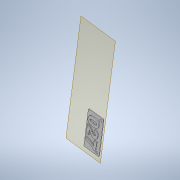
# Autodesk Inventor part: ID Plate
Saved by Autodesk Inventor 2020 (Build 240168000, 168)
## iProperties
Created: 2019-12-31
Part Number: ID Plate
Material: Generic
Document SubType Name: Modeling
Designer: pepd9
Density: 1 g/cm^3
Appearance: Default
Mass: 1.63968 g
Surface Area: 27.9863 cm^2
Volume: 1.63968 cm^3
Author: pepd9
Autodesk Inventor part; units mm, degrees
ref_plane "YZ Plane" through (0, 0, 0) normal (1, 0, 0) x (0, 1, 0)
ref_plane "XZ Plane" through (0, 0, 0) normal (0, 1, 0) x (-1, 0, 0)
ref_plane "XY Plane" through (0, 0, 0) normal (0, 0, 1) x (1, 0, 0)
ref_plane "Work Plane1" through (6.35, -3.5793, 0) normal (0, 0, 1) x (0.9913632, -0.1311451, 0)
sketch "Sketch1" plane through (6.35, -3.5793, 0) normal (0, 0, 1) x (0.9913632, -0.1311451, 0)
  line L0 (9.4349, -35.1273) -> (9.1077, -32.6537) projected
  line L1 (9.1077, -32.6537) -> (11.809, -32.2963) projected
  line L2 (11.809, -32.2963) -> (11.8581, -32.8269) projected
  line L3 (11.8581, -32.8269) -> (12.0044, -33.5342) projected
  spline S0 degree 2 poles (12.0044, -33.5342) (12.2496, -34.5127) (12.9939, -35.3621) (13.7166, -35.5719) knots 0 0 0 1 2 2 2 projected
  line L4 (13.7166, -35.5719) -> (14.274, -35.6456) projected
  line L5 (14.274, -35.6456) -> (14.6409, -38.4193) projected
  line L6 (14.6409, -38.4193) -> (0.7619, -40.2553) projected
  line L7 (0.7619, -40.2553) -> (0.2443, -36.3431) projected
  line L8 (0.2443, -36.3431) -> (9.4349, -35.1273) projected
  line L9 (-0.9482, -27.3284) -> (-1.4726, -23.3645) projected
  line L10 (-1.4726, -23.3645) -> (12.4065, -21.5284) projected
  line L11 (12.4065, -21.5284) -> (13.1225, -26.9414) projected
  spline S1 degree 2 poles (13.1225, -26.9414) (13.3717, -28.825) (11.9849, -30.9988) (10.2534, -31.5228) knots 0 0 0 1 2 2 2 projected
  spline S2 degree 2 poles (10.2534, -31.5228) (9.6848, -31.6822) (9.2839, -31.7563) (9.1286, -31.7769) knots 0 0 0 1 2 2 2 projected
  spline S3 degree 2 poles (9.1286, -31.7769) (7.1725, -32.0356) (4.658, -29.904) (4.3718, -27.7409) knots 0 0 0 1 2 2 2 projected
  line L12 (4.3718, -27.7409) -> (4.2267, -26.6439) projected
  line L13 (4.2267, -26.6439) -> (-0.9482, -27.3284) projected
  line L14 (-4.2533, -2.344) -> (-4.7325, 1.2784) projected
  line L15 (-4.7325, 1.2784) -> (9.1465, 3.1145) projected
  line L16 (9.1465, 3.1145) -> (9.8448, -2.1639) projected
  line L17 (9.8448, -2.1639) -> (2.0845, -4.5596) projected
  line L18 (2.0845, -4.5596) -> (10.2008, -4.8549) projected
  line L19 (10.2008, -4.8549) -> (10.9018, -10.154) projected
  line L20 (10.9018, -10.154) -> (-2.9773, -11.99) projected
  line L21 (-2.9773, -11.99) -> (-3.4565, -8.3676) projected
  line L22 (-3.4565, -8.3676) -> (6.1067, -7.1025) projected
  line L23 (6.1067, -7.1025) -> (-3.6564, -6.8565) projected
  line L24 (-3.6564, -6.8565) -> (-4.0562, -3.8344) projected
  line L25 (-4.0562, -3.8344) -> (5.3099, -1.0789) projected
  line L26 (5.3099, -1.0789) -> (-4.2533, -2.344) projected
  line L27 (-6.2934, 13.0772) -> (-6.8178, 17.0412) projected
  line L28 (-6.8178, 17.0412) -> (7.0613, 18.8772) projected
  line L29 (7.0613, 18.8772) -> (7.7774, 13.4643) projected
  spline S4 degree 2 poles (7.7774, 13.4643) (8.0266, 11.5806) (6.6397, 9.4068) (4.9082, 8.8829) knots 0 0 0 1 2 2 2 projected
  spline S5 degree 2 poles (4.9082, 8.8829) (4.3396, 8.7234) (3.9387, 8.6493) (3.7835, 8.6288) knots 0 0 0 1 2 2 2 projected
  spline S6 degree 2 poles (3.7835, 8.6288) (1.8273, 8.37) (-0.6872, 10.5016) (-0.9734, 12.6647) knots 0 0 0 1 2 2 2 projected
  line L30 (-0.9734, 12.6647) -> (-1.1185, 13.7618) projected
  line L31 (-1.1185, 13.7618) -> (-6.2934, 13.0772) projected
  line L32 (-8.8852, 32.6694) -> (-9.4096, 36.6333) projected
  line L33 (-9.4096, 36.6333) -> (4.4695, 38.4694) projected
  line L34 (4.4695, 38.4694) -> (5.1856, 33.0564) projected
  spline S7 degree 2 poles (5.1856, 33.0564) (5.4348, 31.1728) (4.0479, 28.999) (2.3164, 28.475) knots 0 0 0 1 2 2 2 projected
  spline S8 degree 2 poles (2.3164, 28.475) (1.7478, 28.3156) (1.3469, 28.2415) (1.1917, 28.2209) knots 0 0 0 1 2 2 2 projected
  spline S9 degree 2 poles (1.1917, 28.2209) (-0.7645, 27.9622) (-3.279, 30.0938) (-3.5652, 32.2569) knots 0 0 0 1 2 2 2 projected
  line L35 (-3.5652, 32.2569) -> (-3.7103, 33.3539) projected
  line L36 (-3.7103, 33.3539) -> (-8.8852, 32.6694) projected
  line L37 (-6.9369, 17.9416) -> (-8.0596, 26.4284) projected
  line L38 (-8.0596, 26.4284) -> (5.8195, 28.2645) projected
  line L39 (5.8195, 28.2645) -> (6.923, 19.9225) projected
  line L40 (6.923, 19.9225) -> (3.7146, 19.4981) projected
  line L41 (3.7146, 19.4981) -> (3.1354, 23.8761) projected
  line L42 (3.1354, 23.8761) -> (1.0655, 23.6022) projected
  line L43 (1.0655, 23.6022) -> (1.609, 19.4934) projected
  line L44 (1.609, 19.4934) -> (-1.4649, 19.0867) projected
  line L45 (-1.4649, 19.0867) -> (-2.0084, 23.1956) projected
  line L46 (-2.0084, 23.1956) -> (-4.3268, 22.8889) projected
  line L47 (-4.3268, 22.8889) -> (-3.7284, 18.366) projected
  line L48 (-3.7284, 18.366) -> (-6.9369, 17.9416) projected
  line L49 (-2.3023, -17.0925) -> (-2.7993, -13.3355) projected
  line L50 (-2.7993, -13.3355) -> (11.0798, -11.4995) projected
  line L51 (11.0798, -11.4995) -> (11.5768, -15.2564) projected
  line L52 (11.5768, -15.2564) -> (4.8598, -16.145) projected
  line L53 (4.8598, -16.145) -> (8.406, -17.3187) projected
  line L54 (8.406, -17.3187) -> (8.9249, -21.2413) projected
  line L55 (8.9249, -21.2413) -> (4.2393, -19.0178) projected
  line L56 (4.2393, -19.0178) -> (-1.5205, -23.0022) projected
  line L57 (-1.5205, -23.0022) -> (-2.0504, -18.9968) projected
  line L58 (-2.0504, -18.9968) -> (1.2432, -16.9078) projected
  line L59 (1.2432, -16.9078) -> (0.4818, -16.7242) projected
  line L60 (0.4818, -16.7242) -> (-2.3023, -17.0925) projected
  line L61 (20, -51) -> (-3, -51)
  line L62 (-3, -51) -> (-3, -104)
  line L63 (-3, -104) -> (20, -104)
  line L64 (20, -104) -> (20, -51)
  circle A0 centre (16.3103, -49.711) radius 1.95 projected
  circle A1 centre (-20.0656, -79.7409) radius 1.95 projected
  circle A2 centre (-37.1145, 49.1363) radius 1.95 projected
  line L65 (11.0027, -81.1536) -> (12.4808, -77.5789) projected
  line L66 (7.1679, -81.6609) -> (11.0027, -81.1536) projected
  line L67 (4.8111, -78.5935) -> (7.1679, -81.6609) projected
  line L68 (6.2892, -75.0188) -> (4.8111, -78.5935) projected
  line L69 (10.124, -74.5115) -> (6.2892, -75.0188) projected
  line L70 (12.4808, -77.5789) -> (10.124, -74.5115) projected
  line L71 (2.8138, -48.7477) -> (1.3358, -52.3224) projected
  line L72 (6.6487, -48.2404) -> (2.8138, -48.7477) projected
  line L73 (9.0054, -51.3078) -> (6.6487, -48.2404) projected
  line L74 (7.5273, -54.8825) -> (9.0054, -51.3078) projected
  line L75 (3.6925, -55.3898) -> (7.5273, -54.8825) projected
  line L76 (1.3358, -52.3224) -> (3.6925, -55.3898) projected
  line L77 (9.7896, -71.9835) -> (11.2677, -68.4088) projected
  line L78 (5.9548, -72.4908) -> (9.7896, -71.9835) projected
  line L79 (3.598, -69.4234) -> (5.9548, -72.4908) projected
  line L80 (5.0761, -65.8487) -> (3.598, -69.4234) projected
  line L81 (8.9109, -65.3414) -> (5.0761, -65.8487) projected
  line L82 (11.2677, -68.4088) -> (8.9109, -65.3414) projected
  line L83 (8.5514, -92.1198) -> (7.0733, -95.6945) projected
  line L84 (12.3863, -91.6125) -> (8.5514, -92.1198) projected
  line L85 (14.743, -94.6799) -> (12.3863, -91.6125) projected
  line L86 (13.2649, -98.2547) -> (14.743, -94.6799) projected
  line L87 (9.4301, -98.762) -> (13.2649, -98.2547) projected
  line L88 (7.0733, -95.6945) -> (9.4301, -98.762) projected
  circle A3 centre (-24, -50) radius 1.95 projected
  line L89 (-23.7833, -80.2327) -> (-27.715, -50.5115) projected
  arc A4 (-23.7833, -80.2327) -> (-21.1747, -83.3231) centre (-20.0656, -79.7409) ccw projected
  line L90 (7.3797, -99.9093) -> (-21.1747, -83.3231) projected
  arc A5 (7.3797, -99.9093) -> (7.8548, -100.0043) centre (7.7565, -99.2608) ccw projected
  line L91 (25.6777, -97.6465) -> (7.8548, -100.0043) projected
  arc A6 (25.6777, -97.6465) -> (26.3228, -96.8047) centre (25.5793, -96.903) ccw projected
  line L92 (8.768, 35.8971) -> (26.3228, -96.8047) projected
  arc A7 (8.768, 35.8971) -> (5.0328, 42.3573) centre (-0.8978, 34.6184) ccw projected
  line L93 (-5.2293, 50.2216) -> (5.0328, 42.3573) projected
  arc A8 (-5.2293, 50.2216) -> (-12.4386, 52.1485) centre (-11.1599, 42.4827) ccw projected
  line L94 (-13.3095, 52.0332) -> (-12.4386, 52.1485) projected
  line L95 (-37.6265, 52.8512) -> (-13.3095, 52.0332) projected
  arc A9 (-37.6265, 52.8512) -> (-40.8346, 48.6639) centre (-37.1145, 49.1363) ccw projected
  line L96 (-26.3408, 0.1259) -> (-40.8346, 48.6639) projected
  line L97 (-27.715, -50.5115) -> (-26.3408, 0.1259) projected
  circle A10 centre (22.2118, -94.3224) radius 1.95 projected
  point P0 (-6.7645, 2.7156)
  point P1 (1.0219, -104)
  point P2 (20, -103)
  dimension "d0" = 23
  dimension "d1" = 53
  constraints: 8 end point, 2 parallel, 2 point on line, 1 horizontal, 1 perpendicular
  measures "d0" distance of L62.end L63.end
  measures "d1" distance of L63.end L61.start
extrude "Extrusion1" add sketch "Sketch1" along normal blind 1 contours L64 L91 A5 L90 L62 L61 L71 L76 L75 L74 L73 A0 | A0 L61 | L64 L63 L62 L90 A5 L91 | L73 L74 L75 L76 L71 L61 | L66 L67 L68 L69 L70 L65 | L78 L79 L80 L81 L82 L77 | L84 L85 L86 L87 L88 L83 picked at (16.6806, -51.1045)
fillet "Fillet1" radius 1 4 edges at (-3.3125, -53.7454, 0.5) (-10.2632, -106.2877, 0.5) (12.5381, -109.304, 0.5) (19.4888, -56.7617, 0.5)
sketch "Sketch2" plane through (6.35, -3.5793, 1) normal (0, 0, 1) x (0.9913632, -0.1311451, 0)
  line L0 (15.4266, -55.1181) -> (15.4266, -70.8864) construction
  line L1 (15.4266, -70.8864) -> (9.1495, -70.8864) construction
  line L2 (9.1495, -70.8864) -> (9.1495, -55.1181) construction
  line L3 (9.1495, -55.1181) -> (15.4266, -55.1181) construction
  spline S0 degree 2 poles (7.2188, -56.0421) (11.777, -56.0421) (15.4266, -59.3222) (15.4266, -62.6792) knots 0 0 0 1 2 2 2
  spline S1 degree 2 poles (15.4266, -62.6792) (15.4266, -64.2962) (14.6259, -66.3597) (13.3477, -67.6687) (11.9464, -68.4232) (11.007, -68.6542) knots 0 0 0 1 2 3 4 4 4
  spline S2 degree 2 poles (11.007, -68.6542) (9.2207, -69.1008) (7.2649, -69.1008) knots 0 0 0 1 1 1
  spline S3 degree 2 poles (7.2649, -69.1008) (2.9069, -69.1008) (-1.1277, -66.1595) (-1.1277, -62.556) knots 0 0 0 1 2 2 2
  spline S4 degree 2 poles (-1.1277, -62.556) (-1.1277, -60.5387) (0.1658, -58.0594) (1.4132, -57.2586) knots 0 0 0 1 2 2 2
  spline S5 degree 2 poles (1.4132, -57.2586) (2.2909, -56.6889) (5.3554, -56.0421) (7.2188, -56.0421) knots 0 0 0 1 2 2 2
  spline S6 degree 2 poles (7.2034, -60.4463) (4.1389, -60.4463) (1.906, -61.5243) (1.906, -62.5407) knots 0 0 0 1 2 2 2
  spline S7 degree 2 poles (1.906, -62.5407) (1.906, -63.2182) (2.8607, -64.2192) (4.9088, -64.6812) (7.0802, -64.6812) knots 0 0 0 1 2 3 3 3
  spline S8 degree 2 poles (7.0802, -64.6812) (10.2678, -64.6812) (12.47, -63.6032) (12.47, -62.5253) knots 0 0 0 1 2 2 2
  spline S9 degree 2 poles (12.47, -62.5253) (12.47, -61.4319) (10.237, -60.4463) (7.2034, -60.4463) knots 0 0 0 1 2 2 2
  line L4 (-0.8505, -83.9612) -> (-0.8505, -70.6253)
  spline S10 degree 2 poles (-0.8505, -70.6253) (1.1206, -70.8563) (4.6008, -73.1817) (6.9724, -76.3847) knots 0 0 0 1 2 2 2
  spline S11 degree 2 poles (6.9724, -76.3847) (8.4199, -78.3251) (9.929, -79.4184) (10.6066, -79.4184) knots 0 0 0 1 2 2 2
  spline S12 degree 2 poles (10.6066, -79.4184) (11.3458, -79.4184) (12.3776, -78.3405) (12.3776, -77.5243) knots 0 0 0 1 2 2 2
  spline S13 degree 2 poles (12.3776, -77.5243) (12.3776, -76.6619) (11.315, -75.584) (9.9598, -75.3992) knots 0 0 0 1 2 2 2
  line L5 (9.9598, -75.3992) -> (10.314, -70.9487)
  spline S14 degree 2 poles (10.314, -70.9487) (12.1928, -71.2105) (14.3025, -72.6119) (15.4266, -75.1528) (15.4266, -77.4011) knots 0 0 0 1 2 3 3 3
  spline S15 degree 2 poles (15.4266, -77.4011) (15.4266, -79.7418) (14.3487, -82.3597) (12.1466, -83.8535) (10.7606, -83.8535) knots 0 0 0 1 2 3 3 3
  spline S16 degree 2 poles (10.7606, -83.8535) (9.2977, -83.8535) (6.6336, -82.1441) (5.032, -79.8804) knots 0 0 0 1 2 2 2
  spline S17 degree 2 poles (5.032, -79.8804) (4.1081, -78.5407) (3.3689, -77.6321) (2.7683, -77.0161) knots 0 0 0 1 2 2 2
  line L6 (2.7683, -77.0161) -> (2.7683, -83.9612)
  line L7 (2.7683, -83.9612) -> (-0.8505, -83.9612)
  line L8 (15.1495, -85.9632) -> (15.1495, -98.9295)
  line L9 (15.1495, -98.9295) -> (12.1466, -98.9295)
  spline S18 degree 2 poles (12.1466, -98.9295) (10.622, -97.2355) (8.8357, -96.1114) knots 0 0 0 1 1 1
  spline S19 degree 2 poles (8.8357, -96.1114) (6.6798, -94.7408) (4.0311, -93.9401) knots 0 0 0 1 1 1
  spline S20 degree 2 poles (4.0311, -93.9401) (1.9675, -93.3087) (-0.8505, -93.0931) knots 0 0 0 1 1 1
  line L10 (-0.8505, -93.0931) -> (-0.8505, -88.6581)
  spline S21 degree 2 poles (-0.8505, -88.6581) (3.0609, -89.1817) (8.3737, -91.43) (11.392, -93.8631) knots 0 0 0 1 2 2 2
  line L11 (11.392, -93.8631) -> (11.392, -85.9632)
  line L12 (11.392, -85.9632) -> (15.1495, -85.9632)
  point P0 (-6.7645, 2.7156)
  constraints: 2 other
extrude "Extrusion2" add sketch "Sketch2" along normal blind 1
sketch "Sketch3" plane through (6.35, -3.5793, 1) normal (0, 0, 1) x (0.9913632, -0.1311451, 0)
  arc A0 (19.4855, -94.683) -> (21.161, -96.8637) centre (22.2118, -94.3224) ccw construction
  arc A1 (20.5363, -92.1417) -> (19.4855, -94.683) centre (22.2118, -94.3224) ccw construction
  arc A2 (23.2626, -91.781) -> (20.5363, -92.1417) centre (22.2118, -94.3224) ccw construction
  arc A3 (24.938, -93.9617) -> (23.2626, -91.781) centre (22.2118, -94.3224) ccw construction
  arc A4 (23.8872, -96.503) -> (24.938, -93.9617) centre (22.2118, -94.3224) ccw construction
  arc A5 (21.161, -96.8637) -> (23.8872, -96.503) centre (22.2118, -94.3224) ccw construction
  arc A6 (21.0223, -95.2362) -> (20.7342, -94.0639) centre (22.2118, -94.3224) ccw construction
  arc A7 (20.7342, -94.0639) -> (21.0223, -95.2362) centre (22.2118, -94.3224) ccw construction
  arc A8 (14.6348, -47.5303) -> (13.584, -50.0717) centre (16.3103, -49.711) ccw construction
  arc A9 (17.361, -47.1697) -> (14.6348, -47.5303) centre (16.3103, -49.711) ccw construction
  arc A10 (19.0365, -49.3504) -> (17.361, -47.1697) centre (16.3103, -49.711) ccw construction
  arc A11 (17.9857, -51.8917) -> (19.0365, -49.3504) centre (16.3103, -49.711) ccw construction
  arc A12 (15.2595, -52.2523) -> (17.9857, -51.8917) centre (16.3103, -49.711) ccw construction
  arc A13 (13.584, -50.0717) -> (15.2595, -52.2523) centre (16.3103, -49.711) ccw construction
  arc A14 (14.9241, -49.1379) -> (15.7953, -48.3022) centre (16.3103, -49.711) ccw construction
  arc A15 (15.7953, -48.3022) -> (14.9241, -49.1379) centre (16.3103, -49.711) ccw construction
  line L0 (20, -103) -> (20, -52) projected
  point P0 (-6.7645, 2.7156)
  point P1 (16.5, -55)
  point P2 (16.5, -100)
  point P3 (20, -77.5)
  dimension "d14" = 45
  dimension "d15" = 3.5
  dimension "d16" = 22.5
  constraints: 1 midpoint, 1 vertical alignment
  measures "d14" distance of point (16.5, -55) point (16.5, -100)
  measures "d15" distance from line of L0 point (16.5, -55)
  measures "d16" vertical distance of point (16.5, -100) point (20, -77.5)
hole "Hole1" at (15.4945, -60.2682, 1) at (9.593, -104.8795, 1) direction (0, 0, -1) diameter 3.4 end through all clearance for "Socket Head Cap Screw" size "M3" standard "Ansi Metric M Profile"
sketch "Sketch4" plane through (6.35, -3.5793, 1) normal (0, 0, 1) x (0.9913632, -0.1311451, 0)
  circle A0 centre (16.5, -55) radius 1.7 projected
  circle A1 centre (16.5, -100) radius 1.7 projected
  arc A2 (20, -52) -> (19, -51) centre (19, -52) ccw projected
  line L0 (19, -51) -> (-2, -51) projected
  arc A3 (-2, -51) -> (-3, -52) centre (-2, -52) ccw projected
  line L1 (-3, -52) -> (-3, -103) projected
  arc A4 (-3, -103) -> (-2, -104) centre (-2, -103) ccw projected
  line L2 (-2, -104) -> (19, -104) projected
  arc A5 (19, -104) -> (20, -103) centre (19, -103) ccw projected
  line L3 (20, -103) -> (20, -52) projected
  line L4 (15.1495, -98.9295) -> (12.1466, -98.9295) projected
  line L5 (-0.8505, -93.0931) -> (-0.8505, -88.6581) projected
  line L6 (11.392, -93.8631) -> (11.392, -85.9632) projected
  line L7 (11.392, -85.9632) -> (15.1495, -85.9632) projected
  line L8 (15.1495, -85.9632) -> (15.1495, -98.9295) projected
  line L9 (9.9598, -75.3992) -> (10.314, -70.9487) projected
  line L10 (2.7683, -77.0161) -> (2.7683, -83.9612) projected
  line L11 (2.7683, -83.9612) -> (-0.8505, -83.9612) projected
  line L12 (-0.8505, -83.9612) -> (-0.8505, -70.6253) projected
  point P0 (-6.7645, 2.7156)
  constraints: 18 other
hole "Hole2" at (9.593, -104.8795, 1) direction (0, 0, 1) diameter 3.2 end through all counterbore diameter 6.5 counterbore depth 3 clearance for "Socket Head Cap Screw" size "M3" standard "Ansi Metric M Profile"
body "Solid1"
